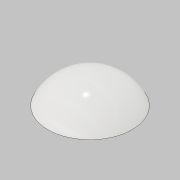
# Autodesk Inventor part: ShellTop
Saved by Autodesk Inventor 2019.2 (Build 232265000, 265)
## iProperties
Created: 2019-02-08
Part Number: ShellTop
Material: ABS-Kunststoff
Document SubType Name: Modeling
Designer: Lion
Density: 1.06 g/cm^3
Appearance: Weiß
Author: Lion
## iProperties of the stored document ShellTop_3D-Druck.ipt
Created: 2019-04-11
Part Number: ShellTop_3D-Druck
Material: Generisch
Document SubType Name: Modeling
Designer: Lion
Density: 1 g/cm^3
Appearance: Vorgabe
Author: Lion
Autodesk Inventor part; units mm, degrees
ref_plane "YZ Plane" through (0, 0, 0) normal (1, 0, 0) x (0, 1, 0)
ref_plane "XZ Plane" through (0, 0, 0) normal (0, 1, 0) x (-1, 0, 0)
derived "ShellLower.ipt"
sketch "Skizze1" plane through (0, 0, 0) normal (0, 1, 0) x (-1, 0, 0)
  arc A0 (-60, 0) -> (60, 0) centre (0, 0) ccw
  arc A1 (-62, 0) -> (62, 0) centre (0, 0) ccw
  line L0 (62, 0) -> (-62, 0)
  arc A2 (60, 0) -> (-60, 0) centre (0, 0) ccw construction
  arc A3 (62, 0) -> (-62, 0) centre (0, 0) ccw construction
  dimension "d1" = 120
  dimension "d2" = 2
  constraints: 8 point on circle, 4 centre point, 2 coincident, 2 end point, 2 point on line, 1 horizontal, 1 midpoint
  measures "d1" diameter of A0
  measures "d2" radial gap between concentric circles of A1 A0
revolve "Umdrehung1" add sketch "Skizze1" angle 180 about axis through (-62, 0, 0) along (1, 0, 0) contours A0 L0 A1
sketch "Skizze3" plane through (0, 0, 0) normal (0, -1, 0) x (1, 0, 0)
  circle A0 centre (0, 0) radius 60 construction
  line L0 (57, 1.5) -> (60, 1.5)
  line L1 (60, 1.5) -> (60, -1.5)
  line L2 (60, -1.5) -> (57, -1.5)
  line L3 (57, -1.5) -> (57, 1.5)
  line L4 (57, 1.5) -> (60, -1.5) construction
  line L5 (60, 1.5) -> (57, -1.5) construction
  line L6 (0, 0) -> (60, 0) construction
  line L7 (0, 0) -> (0, -60) construction
  point P0 (58.5, 0)
  point P1 (58.5, 0)
  dimension "d16" = 3
  dimension "d17" = 3
  constraints: 16 end point, 3 midpoint, 2 horizontal, 2 parallel, 2 point on circle, 1 perpendicular, 1 point on line, 1 tangent, 1 vertical
  measures "d16" distance of L2.end L0.start
  measures "d17" distance of L1.end L2.end
revolve "Umdrehung2" add sketch "Skizze3" angle 180 about axis through (0, 0, 0) along (0, 0, 1)
sketch "Skizze4" plane through (0, 0, 0) normal (0, -1, 0) x (1, 0, 0)
  line L0 (0, 0) -> (0, -60) construction
  line L1 (0, 0) -> (60, 0) construction
  line L2 (-1.5, -57) -> (1.5, -57)
  line L3 (1.5, -57) -> (1.5, -60)
  line L4 (1.5, -60) -> (-1.5, -60)
  line L5 (-1.5, -60) -> (-1.5, -57)
  line L6 (-1.5, -57) -> (1.5, -60) construction
  line L7 (1.5, -57) -> (-1.5, -60) construction
  arc A0 (-59.9812, -1.5) -> (59.9812, -1.5) centre (0, 0) ccw construction
  point P0 (0, -58.5)
  dimension "d19" = 3
  dimension "d20" = 3
  constraints: 12 end point, 2 midpoint, 2 parallel, 1 horizontal, 1 perpendicular, 1 point on line, 1 tangent
  measures "d19" distance of L2.end L3.end
  measures "d20" distance of L2.start L2.end
revolve "Umdrehung3" add sketch "Skizze4" angle 180 about axis through (0, 0, 0) along (1, 0, 0)
ref_plane "Arbeitsebene1" through (0, 26, 0) normal (0, -1, 0) x (1, 0, 0)
split "Trennen1" plane through (0, 26, 0) removes the side toward (0, -1, 0)
sketch "Skizze2" plane through (0, 26, 0) normal (0, -1, 0) x (1, 0, 0)
  line L0 (3.5, -54.074) -> (-3.5, -54.074)
  line L1 (-3.5, -54.074) -> (-3.5, -46)
  line L2 (-3.5, -46) -> (3.5, -46)
  line L3 (3.5, -46) -> (3.5, -54.074)
  line L4 (3.5, -54.074) -> (-3.5, -46) construction
  line L5 (-3.5, -54.074) -> (3.5, -46) construction
  circle A0 centre (0, 0) radius 54.074 construction
  line L6 (0, -54.074) -> (0, 0) construction
  line L7 (54.074, 3.5) -> (54.074, -3.5)
  line L8 (54.074, -3.5) -> (46, -3.5)
  line L9 (46, -3.5) -> (46, 3.5)
  line L10 (46, 3.5) -> (54.074, 3.5)
  line L11 (54.074, 3.5) -> (46, -3.5) construction
  line L12 (54.074, -3.5) -> (46, 3.5) construction
  line L13 (-3.5, 54.074) -> (3.5, 54.074)
  line L14 (3.5, 54.074) -> (3.5, 46)
  line L15 (3.5, 46) -> (-3.5, 46)
  line L16 (-3.5, 46) -> (-3.5, 54.074)
  line L17 (-3.5, 54.074) -> (3.5, 46) construction
  line L18 (3.5, 54.074) -> (-3.5, 46) construction
  line L19 (-54.074, -3.5) -> (-54.074, 3.5)
  line L20 (-54.074, 3.5) -> (-46, 3.5)
  line L21 (-46, 3.5) -> (-46, -3.5)
  line L22 (-46, -3.5) -> (-54.074, -3.5)
  line L23 (-54.074, -3.5) -> (-46, 3.5) construction
  line L24 (-54.074, 3.5) -> (-46, -3.5) construction
  point P0 (0, -50.037)
  point P1 (0, -50.037)
  point P2 (50.037, 0)
  point P3 (50.037, 0)
  point P4 (54.074, 0)
  point P5 (0, 50.037)
  point P6 (0, 50.037)
  point P7 (0, 54.074)
  point P8 (-50.037, 0)
  point P9 (-50.037, 0)
  point P10 (-54.074, 0)
  dimension "d5" = 46
  dimension "d6" = 7
  dimension "d10" = 360
  constraints: 50 end point, 9 midpoint, 2 horizontal, 2 parallel, 1 perpendicular, 1 point on line, 1 vertical, 1 vertical alignment, 54 other
  measures "d5" distance from line of point (0, 0) L2
  measures "d6" distance between parallel lines of L3 L1
extrude "Extrusion1" add sketch "Skizze2" against normal up to next
extrude "Extrusion2" cut sketch "Skizze2" against normal blind 2
fillet "Rundung1" [suppressed]
equation "\"d1\" = d_inner"
equation "\"d_inner\" = 120"
